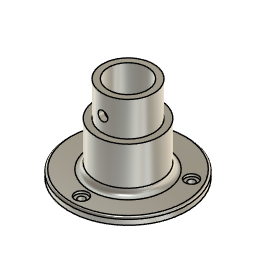
EchoWeather_Main_PipeAdapter_ (Autodesk Fusion 360 design; units mm, degrees)
Autodesk Fusion 360 part; units mm, degrees
sketch "Sketch1" plane through (0, 0, 0) normal (0, 0, 1) x (1, 0, 0)
  circle A0 centre (0, 0) radius 16.51
  circle A1 centre (0, 0) radius 12.7
  circle A2 centre (0, 0) radius 38.1
  dimension "d1" = 33.02
  dimension "d2" = 25.4
  dimension "d3" = 76.2
  constraint coincident A0.centre A1.centre
  constraint concentric A0 A1
  constraint concentric A0 A2
  measures "d1" diameter of A0
  measures "d2" diameter of A1
  measures "d3" diameter of A2
extrude "Extrude1" add sketch "Sketch1" along normal blind 50.8 contours A0
extrude "Extrude2" add sketch "Sketch1" against normal blind 4.572 contours A0 | A2
sketch "Sketch3" plane through (0, 0, 0) normal (0, 0, 1) x (1, 0, 0)
  line L0 (0, 0) -> (0, -39.9504) construction
  line L1 (0, 0) -> (-48.5556, 28.0336) construction
  line L2 (0, 0) -> (38.9341, 22.4786) construction
  circle A0 centre (0, 0) radius 30.1625 construction
  circle A1 centre (0, -30.1625) radius 2.159
  circle A2 centre (-26.1215, 15.0812) radius 2.159
  circle A3 centre (26.1215, 15.0812) radius 2.159
  circle A4 centre (0, -30.1625) radius 4.191
  circle A5 centre (-26.1215, 15.0812) radius 4.191
  circle A6 centre (26.1215, 15.0812) radius 4.191
  dimension "d8" = 120
  dimension "d9" = 120
  dimension "d10" = 60.325
  dimension "d11" = 4.318
  dimension "d12" = 8.382
  constraint coincident L0.start L1.start
  constraint vertical L0
  constraint coincident L0 A1.centre
  constraint coincident A0 A1.centre
  constraint coincident A0 A2.centre
  constraint coincident L1 A2.centre
  constraint coincident L2 A3.centre
  constraint coincident A0 A3.centre
  constraint equal A2 A3
  constraint equal A1 A2
  constraint concentric A1 A4
  constraint concentric A2 A5
  constraint concentric A3 A6
  constraint equal A4 A6
  constraint equal A5 A6
  measures "d8" angle of L0 L2
  measures "d9" angle of L0 L1
  measures "d10" diameter of A0
  measures "d11" diameter of A1
  measures "d12" diameter of A5
extrude "Extrude3" cut sketch "Sketch3" against normal up to surface (4.572 mm away) contours A1 | A2 | A3
extrude "Extrude4" cut sketch "Sketch3" against normal blind 1.5875
sketch "Sketch4" plane through (0, 0, 0) normal (0, 1, 0) x (1, 0, 0)
  line L0 (0, 0) -> (0, -68.6315) construction
  circle A0 centre (0, -38.1) radius 3.1
  line L1 (0, 0) -> (-36.56, 0) construction
  line L2 (-16.51, -50.8) -> (16.51, -50.8) construction
  dimension "d17" = 6.2
  dimension "d19" = 12.7
  constraint coincident L0.start L1.start
  constraint vertical L0
  constraint coincident L0 A0.centre
  constraint perpendicular L0 L1
  measures "d17" diameter of A0
  measures "d19" distance of A0.centre L2
extrude "Extrude5" cut sketch "Sketch4" against normal blind 28.9814
sketch "Sketch5" plane through (0, 0, 0) normal (0, 0, 1) x (-1, 0, 0)
  circle A0 centre (-26.1215, -15.0812) radius 4.191
  circle A1 centre (26.1215, -15.0812) radius 4.191
  circle A2 centre (0, 30.1625) radius 4.191
  circle A3 centre (0, 0) radius 38.1
  circle A4 centre (0, 0) radius 16.51
  circle A5 centre (0, 0) radius 16.51
  circle A6 centre (0, 0) radius 20.574
  dimension "d22" = 41.148
  constraint coincident A3.centre A4.centre
  constraint concentric A5 A6
  measures "d22" diameter of A6
extrude "Extrude6" add sketch "Sketch5" along normal blind 28.575 contours A6
fillet "Fillet1" radius 3.81 1 edges at (19.1817, -7.4399, 0)
fillet "Fillet2" radius 1.27 1 edges at (-35.5217, -13.7775, 0)
